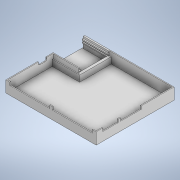
# Autodesk Inventor part: BaseCase
Saved by Autodesk Inventor 2022 (Build 260153070, 153G)
## iProperties
Created: 2021-07-15
Part Number: BaseCase
Material: Generic
Document SubType Name: Modeling
Designer: Eakawit_kor
Density: 1 g/cm^3
Appearance: Default
Author: Eakawit_kor
Autodesk Inventor part; units mm, degrees
ref_plane "YZ Plane" through (0, 0, 0) normal (1, 0, 0) x (0, 1, 0)
ref_plane "XZ Plane" through (0, 0, 0) normal (0, 1, 0) x (-1, 0, 0)
ref_plane "XY Plane" through (0, 0, 0) normal (0, 0, 1) x (1, 0, 0)
sketch "Sketch1" plane through (0, 0, 0) normal (0, 1, 0) x (-1, 0, 0)
  line L0 (0, 0) -> (102, 0)
  line L1 (102, 0) -> (102, -88)
  line L2 (102, -88) -> (0, -88)
  line L3 (0, -88) -> (0, 0)
  dimension "d0" = 102
  dimension "d1" = 88
  constraints: 8 end point, 2 parallel, 1 horizontal, 1 perpendicular
  measures "d0" distance of L0.start L0.end
  measures "d1" distance of L0.end L1.end
extrude "Extrusion1" add sketch "Sketch1" along normal blind 1
sketch "Sketch3" plane through (0, 1, 0) normal (0, 1, 0) x (1, 0, 0)
  line L0 (0, 88) -> (-102, 88) projected
  line L1 (-102, 0) -> (0, 0) projected
  line L2 (-102, 88) -> (0, 88)
  line L3 (0, 88) -> (0, 0)
  line L4 (0, 0) -> (-102, 0)
  line L5 (-102, 0) -> (-102, 88)
  line L6 (-1, 1) -> (-1, 87)
  line L7 (-1, 87) -> (-101, 87)
  line L8 (-101, 87) -> (-101, 1)
  line L9 (-101, 1) -> (-1, 1)
  dimension "d7" = 1
  constraints: 16 end point, 4 parallel, 2 perpendicular, 1 horizontal, 3 other
  measures "d7" distance between parallel lines of L5 L8
extrude "Extrusion3" add sketch "Sketch3" along normal blind 12
sketch "Sketch4" plane through (-102, 0, 0) normal (0, 0, 1) x (1, 0, 0)
  line L0 (101, 13) -> (1, 13) projected
  line L1 (4.398, 13) -> (49.698, 13)
  line L2 (49.698, 13) -> (49.698, 9.6)
  line L3 (49.698, 9.6) -> (4.398, 9.6)
  line L4 (4.398, 9.6) -> (4.398, 13)
  line L5 (52.298, 13) -> (97.598, 13)
  line L6 (97.598, 13) -> (97.598, 9.6)
  line L7 (97.598, 9.6) -> (52.298, 9.6)
  line L8 (52.298, 9.6) -> (52.298, 13)
  line L9 (102, 0) -> (102, 13) projected
  line L10 (0, 0) -> (102, 0) projected
  dimension "d10" = 45.3
  dimension "d11" = 4.402
  dimension "d12" = 2.6
  dimension "d13" = 9.6
  constraints: 16 end point, 4 parallel, 3 point on line, 2 horizontal, 2 perpendicular, 1 collinear
  measures "d10" distance of L6.end L7.end
  measures "d11" distance between parallel lines of L9 L6
  measures "d12" distance between parallel lines of L2 L8
  measures "d13" distance between parallel lines of L10 L7
extrude "Extrusion4" cut sketch "Sketch4" against normal up to surface (1 mm away)
sketch "Sketch5" plane through (0, 0, 0) normal (1, 0, 0) x (0, 0, -1)
  line L0 (7.371, 13) -> (24.671, 13)
  line L1 (24.671, 13) -> (24.671, 9.6)
  line L2 (24.671, 9.6) -> (7.371, 9.6)
  line L3 (7.371, 9.6) -> (7.371, 13)
  line L4 (27.5, 13) -> (50.8, 13)
  line L5 (50.8, 13) -> (50.8, 9.6)
  line L6 (50.8, 9.6) -> (27.5, 9.6)
  line L7 (27.5, 9.6) -> (27.5, 13)
  line L8 (0, 13) -> (88, 13) projected
  line L9 (0, 0) -> (88, 0) projected
  line L10 (0, 13) -> (0, 9.6) projected
  dimension "d16" = 17.3
  dimension "d17" = 23.3
  dimension "d19" = 7.371
  dimension "d20" = 2.829
  constraints: 16 end point, 5 parallel, 2 horizontal, 2 perpendicular, 2 point on line, 1 collinear
  measures "d16" distance of L1.end L2.end
  measures "d17" distance of L5.end L6.end
  measures "d19" distance between parallel lines of L10 L3
  measures "d20" distance between parallel lines of L7 L1
extrude "Extrusion5" cut sketch "Sketch5" against normal up to surface (1 mm away)
sketch "Sketch6" plane through (-102, 0, -88) normal (-1, 0, 0) x (0, 0, 1)
  line L0 (44.58, 11.3) -> (50.68, 11.3) construction
  line L1 (44.58, 9.6) -> (50.68, 9.6)
  arc A0 (42.88, 11.3) -> (44.58, 9.6) centre (44.58, 11.3) ccw
  arc A1 (50.68, 9.6) -> (52.38, 11.3) centre (50.68, 11.3) ccw
  line L2 (87, 1) -> (87, 13) projected
  line L3 (0, 0) -> (88, 0) projected
  line L4 (0, 13) -> (88, 13) projected
  line L5 (87, 13) -> (1, 13) projected
  line L6 (42.88, 13) -> (42.88, 11.3)
  line L7 (52.38, 11.3) -> (52.38, 13)
  line L8 (60.5, 9.6) -> (37.2, 9.6) projected
  line L9 (42.88, 13) -> (52.38, 13)
  point P0 (47.63, 11.3)
  dimension "d24" = 39.37
  dimension "d25" = 9.5
  dimension "d50" = 1.7
  dimension "d51" = 1.7
  dimension "d52" = 1.7
  dimension "d53" = 1.7
  constraints: 12 end point, 4 point on circle, 2 centre point, 2 parallel, 2 point on line, 2 tangent, 1 collinear, 1 midpoint, 1 perpendicular
  measures "d24" distance from line of L2 point (47.63, 11.3)
  measures "d50" distance from line of L8 L0.start
  measures "d51" radius of A0
  measures "d52" radius of A1
  measures "d53" distance of L6.start L6.end
extrude "Extrusion6" cut sketch "Sketch6" against normal up to surface (1 mm away)
sketch "Sketch7" plane through (-102, 0, -88) normal (-1, 0, 0) x (0, 0, 1)
  line L0 (1, 1) -> (87, 1) projected
  line L1 (0, 13) -> (34.7, 13)
  line L2 (34.7, 13) -> (34.7, 1)
  line L3 (34.7, 1) -> (0, 1)
  line L4 (0, 1) -> (0, 13)
  line L5 (0, 13) -> (88, 13) projected
  line L6 (0, 0) -> (0, 13) projected
  point P0 (88, 0)
  dimension "d30" = 34.7
  constraints: 8 end point, 2 collinear, 2 parallel, 1 horizontal, 1 perpendicular, 1 point on line
  measures "d30" distance of L2.end L3.end
extrude "Extrusion7" cut sketch "Sketch7" against normal up to surface (1 mm away)
sketch "Sketch8" plane through (0, 1, 0) normal (0, 1, 0) x (1, 0, 0)
  line L0 (-101, 54.3) -> (-73, 54.3)
  line L1 (-70, 53.4922) -> (-70, 51.3)
  line L2 (-70, 51.3) -> (-101, 51.3)
  line L3 (-101, 51.3) -> (-101, 54.3)
  line L4 (-1, 87) -> (-101, 87) projected
  line L5 (-73, 54.3) -> (-73, 85)
  line L6 (-73, 87) -> (-70, 87)
  line L7 (-70, 87) -> (-70, 53.4922)
  line L8 (-101, 53.3) -> (-101, 1) projected
  line L9 (-102, 53.3) -> (-101, 53.3) projected
  line L10 (-73, 87) -> (-101, 87)
  line L11 (-101, 87) -> (-101, 85)
  line L12 (-101, 85) -> (-73, 85)
  point P0 (0, 0)
  dimension "d33" = 3
  dimension "d34" = 3
  dimension "d38" = 31
  dimension "d39" = 2
  dimension "d40" = 2
  constraints: 20 end point, 4 collinear, 4 parallel, 2 horizontal, 2 perpendicular, 1 point on line
  measures "d33" distance between parallel lines of L2 L0
  measures "d34" distance between parallel lines of L7 L5
  measures "d38" distance between parallel lines of L3 L7
  measures "d39" distance between parallel lines of L9 L2
  measures "d40" distance between parallel lines of L10 L12
extrude "Extrusion8" add sketch "Sketch8" along normal blind 7
sketch "Sketch9" plane through (0, 8, 0) normal (0, 1, 0) x (1, 0, 0)
  line L0 (-101, 53.3) -> (-72, 53.3)
  line L1 (-72, 53.3) -> (-72, 52.3)
  line L2 (-72, 52.3) -> (-101, 52.3)
  line L3 (-101, 52.3) -> (-101, 53.3)
  line L4 (-73, 54.3) -> (-101, 54.3) projected
  line L5 (-101, 51.3) -> (-70, 51.3) projected
  line L6 (-101, 85) -> (-101, 88) projected
  line L7 (-101, 87) -> (-72, 87)
  line L8 (-72, 87) -> (-72, 86.3)
  line L9 (-72, 86.3) -> (-101, 86.3)
  line L10 (-101, 86.3) -> (-101, 87)
  line L11 (-101, 87) -> (-70, 87) projected
  line L12 (-73, 85) -> (-73, 54.3) projected
  point P0 (0, 0)
  point P1 (-101, 86.3)
  dimension "d41" = 1
  dimension "d42" = 1
  dimension "d45" = 0.7
  dimension "d46" = 1
  constraints: 16 end point, 4 parallel, 2 collinear, 2 horizontal, 2 perpendicular, 1 point on line
  measures "d41" distance between parallel lines of L4 L0
  measures "d42" distance between parallel lines of L5 L2
  measures "d45" distance between parallel lines of L7 L9
  measures "d46" distance between parallel lines of L8 L12
extrude "Extrusion9" add sketch "Sketch9" along normal up to surface (5 mm away)
sketch "Sketch10" plane through (-101, 1, -54.3) normal (-1, 0, 0) x (0, 0, 1)
  line L0 (1, 0) -> (1, 7) projected
  line L1 (53.3, 0) -> (-32.7, 0) projected
  line L2 (1, 6) -> (-32, 6)
  line L3 (-32, 6) -> (-32, 0)
  line L4 (-32, 0) -> (1, 0)
  line L5 (1, 0) -> (1, 6)
  line L6 (-32, 7) -> (-32, 12) projected
  line L7 (-30.7, 7) -> (0, 7) projected
  point P0 (54.3, -1)
  point P1 (1, 10)
  dimension "d47" = 1
  constraints: 8 end point, 2 parallel, 2 point on line, 1 collinear, 1 horizontal, 1 perpendicular
  measures "d47" distance between parallel lines of L2 L7
extrude "Extrusion10" cut sketch "Sketch10" against normal up to surface (28 mm away)
sketch "Sketch11" plane through (-101, 8, -54.3) normal (-1, 0, 0) x (0, 0, 1)
  line L0 (1, 5) -> (1, -7) projected
  line L1 (1, 1.6) -> (0, 1.6)
  line L2 (0, 1.6) -> (0, 2.9)
  line L3 (0, 2.9) -> (1, 2.9)
  line L4 (1, 2.9) -> (1, 1.6)
  line L5 (-32, 0) -> (-32, 5) projected
  line L6 (-32, 1.6) -> (-30.7, 1.6)
  line L7 (-30.7, 1.6) -> (-30.7, 2.9)
  line L8 (-30.7, 2.9) -> (-32, 2.9)
  line L9 (-32, 2.9) -> (-32, 1.6)
  line L10 (-32, 0) -> (-30.7, 0) projected
  line L11 (-30.7, -1) -> (-30.7, 0) projected
  line L12 (0, -1) -> (0, 0) projected
  point P0 (54.3, -8)
  point P1 (1, 2.9)
  point P2 (-32, 2.9)
  dimension "d54" = 1.6
  constraints: 16 end point, 4 parallel, 4 point on line, 3 equal length, 2 collinear, 2 horizontal, 2 perpendicular
  measures "d54" distance between parallel lines of L10 L6
extrude "Extrusion11" add sketch "Sketch11" against normal up to surface (29 mm away)
body "Solid1"
